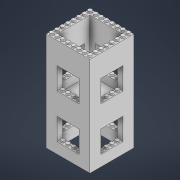
# Autodesk Inventor part: 110033226_ipt_28_城堡四圓塔
Saved by Autodesk Inventor 2022 (Build 260153000, 153)
## iProperties
Created: 2022-06-24
Part Number: 110033226_ipt_28_城堡四圓塔
Material: 一般
Document SubType Name: Modeling
Designer: User
Density: 1 g/cm^3
Appearance: 預設
Author: User
Autodesk Inventor part; units mm, degrees
ref_plane "YZ Plane" through (0, 0, 0) normal (1, 0, 0) x (0, 1, 0)
ref_plane "XZ Plane" through (0, 0, 0) normal (0, 1, 0) x (-1, 0, 0)
ref_plane "XY Plane" through (0, 0, 0) normal (0, 0, 1) x (1, 0, 0)
sketch "草圖1" plane through (0, 0, 0) normal (0, 1, 0) x (-1, 0, 0)
  line L0 (20, 20) -> (-20, 20)
  line L1 (-20, 20) -> (-20, -20)
  line L2 (-20, -20) -> (20, -20)
  line L3 (20, -20) -> (20, 20)
  circle A0 centre (17.5, 17.5) radius 1.7
  circle A1 centre (17.5, 12.5) radius 1.7
  circle A2 centre (17.5, 7.5) radius 1.7
  circle A3 centre (17.5, 2.5) radius 1.7
  circle A4 centre (17.5, -2.5) radius 1.7
  circle A5 centre (17.5, -7.5) radius 1.7
  circle A6 centre (17.5, -12.5) radius 1.7
  circle A7 centre (17.5, -17.5) radius 1.7
  circle A8 centre (12.5, 17.5) radius 1.7
  circle A9 centre (12.5, 12.5) radius 1.7
  circle A10 centre (12.5, 7.5) radius 1.7
  circle A11 centre (12.5, 2.5) radius 1.7
  circle A12 centre (12.5, -2.5) radius 1.7
  circle A13 centre (12.5, -7.5) radius 1.7
  circle A14 centre (12.5, -12.5) radius 1.7
  circle A15 centre (12.5, -17.5) radius 1.7
  circle A16 centre (7.5, 17.5) radius 1.7
  circle A17 centre (7.5, 12.5) radius 1.7
  circle A18 centre (7.5, 7.5) radius 1.7
  circle A19 centre (7.5, 2.5) radius 1.7
  circle A20 centre (7.5, -2.5) radius 1.7
  circle A21 centre (7.5, -7.5) radius 1.7
  circle A22 centre (7.5, -12.5) radius 1.7
  circle A23 centre (7.5, -17.5) radius 1.7
  circle A24 centre (2.5, 17.5) radius 1.7
  circle A25 centre (2.5, 12.5) radius 1.7
  circle A26 centre (2.5, 7.5) radius 1.7
  circle A27 centre (2.5, 2.5) radius 1.7
  circle A28 centre (2.5, -2.5) radius 1.7
  circle A29 centre (2.5, -7.5) radius 1.7
  circle A30 centre (2.5, -12.5) radius 1.7
  circle A31 centre (2.5, -17.5) radius 1.7
  circle A32 centre (-2.5, 17.5) radius 1.7
  circle A33 centre (-2.5, 12.5) radius 1.7
  circle A34 centre (-2.5, 7.5) radius 1.7
  circle A35 centre (-2.5, 2.5) radius 1.7
  circle A36 centre (-2.5, -2.5) radius 1.7
  circle A37 centre (-2.5, -7.5) radius 1.7
  circle A38 centre (-2.5, -12.5) radius 1.7
  circle A39 centre (-2.5, -17.5) radius 1.7
  circle A40 centre (-7.5, 17.5) radius 1.7
  circle A41 centre (-7.5, 12.5) radius 1.7
  circle A42 centre (-7.5, 7.5) radius 1.7
  circle A43 centre (-7.5, 2.5) radius 1.7
  circle A44 centre (-7.5, -2.5) radius 1.7
  circle A45 centre (-7.5, -7.5) radius 1.7
  circle A46 centre (-7.5, -12.5) radius 1.7
  circle A47 centre (-7.5, -17.5) radius 1.7
  circle A48 centre (-12.5, 17.5) radius 1.7
  circle A49 centre (-12.5, 12.5) radius 1.7
  circle A50 centre (-12.5, 7.5) radius 1.7
  circle A51 centre (-12.5, 2.5) radius 1.7
  circle A52 centre (-12.5, -2.5) radius 1.7
  circle A53 centre (-12.5, -7.5) radius 1.7
  circle A54 centre (-12.5, -12.5) radius 1.7
  circle A55 centre (-12.5, -17.5) radius 1.7
  circle A56 centre (-17.5, 17.5) radius 1.7
  circle A57 centre (-17.5, 12.5) radius 1.7
  circle A58 centre (-17.5, 7.5) radius 1.7
  circle A59 centre (-17.5, 2.5) radius 1.7
  circle A60 centre (-17.5, -2.5) radius 1.7
  circle A61 centre (-17.5, -7.5) radius 1.7
  circle A62 centre (-17.5, -12.5) radius 1.7
  circle A63 centre (-17.5, -17.5) radius 1.7
  line L4 (15, 15) -> (-15, 15)
  line L5 (-15, 15) -> (-15, -15)
  line L6 (-15, -15) -> (15, -15)
  line L7 (15, -15) -> (15, 15)
  point P0 (0, 0)
  point P1 (20, 0)
  point P2 (0, -20)
  dimension "d0" = 40
  dimension "d1" = 40
  dimension "d2" = 3.4
  dimension "d3" = 2.5
  dimension "d4" = 2.5
  dimension "d7" = 5
  dimension "d10" = 5
  dimension "d31" = 5
  constraints: 64 centre point, 16 end point, 4 parallel, 2 horizontal, 2 midpoint, 2 perpendicular, 1 horizontal alignment, 1 vertical, 1 vertical alignment, 129 other
  measures "d0" distance of L2.end L1.end
  measures "d1" distance of L1.end L0.end
  measures "d2" diameter of A0
  measures "d3" distance from line of L3 A0.centre
  measures "d4" distance from line of L0 A0.centre
  measures "d7" distance of A0.centre A1.centre
  measures "d10" distance of A0.centre A8.centre
  measures "d31" distance between parallel lines of L3 L7
extrude "擠出4" add sketch "草圖1" along normal blind 90 contours L3 L2 L1 L0 | A0 | A1 | A2 | A3 | A4 | A5 | A6 | A7 | A8 | A15 | A16 | A23 | A24 | A31 | A32 | A39 | A40 | A47 | A48 | A55 | A56 | A57 | A58 | A59 | A60 | A61 | A62 | A63
extrude "擠出5" cut sketch "草圖1" along normal blind 1.5 contours A0 | A1 | A2 | A3 | A4 | A5 | A6 | A7 | A8 | A15 | A16 | A23 | A24 | A31 | A32 | A39 | A40 | A47 | A48 | A55 | A56 | A57 | A58 | A59 | A60 | A61 | A62 | A63
sketch "草圖3" plane through (0, 90, 0) normal (0, 1, 0) x (1, 0, 0)
  circle A0 centre (-17.5, 17.5) radius 1.7 projected
  point P0 (0, 0)
extrude "擠出6" add sketch "草圖3" along normal blind 1.5
pattern_linear "矩形陣列3" count 8 spacing 5 along (1, 0, 0) count 2 spacing 35 along (0, 0, 1) of "擠出6"
sketch "草圖4" plane through (0, 90, 0) normal (0, 1, 0) x (1, 0, 0)
  circle A0 centre (-17.5, 12.5) radius 1.7 projected
  point P0 (0, 0)
extrude "擠出7" add sketch "草圖4" along normal blind 1.5
pattern_linear "矩形陣列4" count 6 spacing 5 along (0, 0, 1) count 2 spacing 35 along (1, 0, 0) of "擠出7"
sketch "草圖5" plane through (20, 0, 20) normal (1, 0, 0) x (0, 0, -1)
  line L0 (0, 0) -> (40, 0) projected
  line L1 (40, 0) -> (40, 90) projected
  line L2 (0, 90) -> (40, 90) projected
  line L3 (0, 0) -> (0, 90) projected
  line L4 (10, 30) -> (30, 30)
  line L5 (30, 30) -> (30, 10)
  line L6 (30, 10) -> (10, 10)
  line L7 (10, 10) -> (10, 30)
  line L8 (10, 70) -> (30, 70)
  line L9 (30, 70) -> (30, 50)
  line L10 (30, 50) -> (10, 50)
  line L11 (10, 50) -> (10, 70)
  point P0 (20, 0)
  point P1 (20, 30)
  point P2 (20, 90)
  point P3 (20, 70)
  dimension "d52" = 20
  dimension "d53" = 20
  dimension "d54" = 10
  dimension "d57" = 40
  constraints: 16 end point, 2 midpoint, 2 parallel, 1 horizontal, 1 perpendicular, 1 vertical, 1 vertical alignment, 9 other
  measures "d52" distance of L5.end L6.end
  measures "d53" distance of L4.end L5.end
  measures "d54" distance between parallel lines of L0 L6
  measures "d57" distance of L4.start L8.start
extrude "擠出8" cut sketch "草圖5" against normal up to surface (5 mm away) contours L4 L5 L6 L7 | L8 L9 L10 L11
pattern_circular "環形陣列1" count 4 over 360 about axis through (0, -10, 0) along (0, 1, 0) of "擠出8"
ref_plane "工作平面1" through (0, 40, 0) normal (0, -1, 0) x (1, 0, 0)
sketch "草圖6" plane through (0, 40, 0) normal (0, -1, 0) x (1, 0, 0)
  line L0 (15, 15) -> (-15, 15) projected
  line L1 (-15, 15) -> (-15, -15) projected
  line L2 (-15, -15) -> (15, -15) projected
  line L3 (15, -15) -> (15, 15) projected
  line L4 (-20, 20) -> (20, 20) projected
  line L5 (20, 20) -> (20, -20) projected
  line L6 (20, -20) -> (-20, -20) projected
  line L7 (-20, -20) -> (-20, 20) projected
  point P0 (0, 0)
extrude "擠出9" add sketch "草圖6" along normal mid plane 5 contours L3 L2 L1 L0
sketch "草圖7" plane through (-10, 50, 15) normal (0, 1, 0) x (1, 0, 0)
  circle A0 centre (2.5, -2.5) radius 1.7 projected
  point P0 (10, 15)
extrude "擠出10" add sketch "草圖7" along normal blind 1.5
pattern_linear "矩形陣列5" count 4 spacing 5 along (1, 0, 0) of "擠出10"
pattern_circular "環形陣列2" count 4 over 360 about axis through (0, -10, 0) along (0, 1, 0) of "擠出10", "矩形陣列5"
pattern_linear "矩形陣列6" count 2 spacing 40 along (0, -1, 0) of "擠出10", "矩形陣列5", "環形陣列2"
